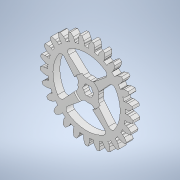
# Autodesk Inventor part: ｍ2歯数25ギア_6
Saved by Autodesk Inventor 2020.2 (Build 242310000, 310)
## iProperties
Created: 2020-03-11
Part Number: ｍ2歯数25ギア_6
Material: アルミニウム 2014-T4
Document SubType Name: Modeling
Designer: aoyam
Density: 2.8 g/cm^3
Appearance: サテン
Mass: 16.0283 g
Surface Area: 48.4557 cm^2
Volume: 5.70401 cm^3
Author: aoyam
Autodesk Inventor part; units mm, degrees
(part 1 of 2)
ref_plane "YZ Plane" through (0, 0, 0) normal (1, 0, 0) x (0, 1, 0)
ref_plane "XZ Plane" through (0, 0, 0) normal (0, 1, 0) x (-1, 0, 0)
ref_plane "XY Plane" through (0, 0, 0) normal (0, 0, 1) x (1, 0, 0)
sketch "スケッチ1" plane through (0, 0, 0) normal (0, 0, 1) x (1, 0, 0)
  arc A0 (2.4204, 26.4789) -> (2.3628, 26.1303) centre (4.6419, 25.9331) ccw
  arc A1 (2.7863, 27.5676) -> (2.4204, 26.4789) centre (8.5404, 25.0277) ccw
  arc A2 (3.906, 29.5327) -> (2.7863, 27.5676) centre (12.7407, 23.1969) ccw
  arc A3 (0.1118, 26.1303) -> (0.0542, 26.4789) centre (-2.1673, 25.9331) ccw
  arc A4 (0.0542, 26.4789) -> (-0.3117, 27.5676) centre (-6.0658, 25.0277) ccw
  arc A5 (-0.3117, 27.5676) -> (-1.4314, 29.5327) centre (-10.2661, 23.1969) ccw
  arc A6 (2.3153, 25.1391) -> (0.1593, 25.1391) centre (1.2373, 2.6649) ccw
  arc A7 (-1.4314, 29.5327) -> (-2.8596, 29.3523) centre (1.2373, 2.6649) ccw
  line L0 (2.3153, 25.1391) -> (2.3628, 26.1303)
  line L1 (0.1593, 25.1391) -> (0.1118, 26.1303)
  arc A8 (-3.5391, 26.0249) -> (-3.5082, 25.6729) centre (-1.2516, 26.0487) ccw
  line L2 (-3.3077, 24.7011) -> (-3.5082, 25.6729)
  arc A9 (-3.4554, 27.1705) -> (-3.5391, 26.0249) centre (2.7495, 26.1414) ccw
  arc A10 (-2.8596, 29.3523) -> (-3.4554, 27.1705) centre (7.2732, 25.4126) ccw
  arc A11 (-3.3077, 24.7011) -> (-5.3959, 24.1649) centre (1.2373, 2.6649) ccw
  line L3 (-5.3959, 24.1649) -> (-5.6884, 25.1131)
  arc A12 (-5.6884, 25.1131) -> (-5.8309, 25.4365) centre (-7.8469, 24.3554) ccw
  arc A13 (-6.4561, 26.4001) -> (-8.0293, 28.0249) centre (-15.0108, 19.691) ccw
  arc A14 (-8.0293, 28.0249) -> (-9.3677, 27.495) centre (1.2373, 2.6649) ccw
  arc A15 (-5.8309, 25.4365) -> (-6.4561, 26.4001) centre (-11.3978, 22.509) ccw
  arc A16 (-9.1985, 24.1032) -> (-9.0809, 23.77) centre (-6.9887, 24.6951) ccw
  line L4 (-8.6451, 22.8785) -> (-9.0809, 23.77)
  arc A17 (-9.4023, 25.2336) -> (-9.1985, 24.1032) centre (-3.1363, 25.7799) ccw
  arc A18 (-9.3677, 27.495) -> (-9.4023, 25.2336) centre (1.4265, 26.199) ccw
  arc A19 (-8.6451, 22.8785) -> (-10.5343, 21.8399) centre (1.2373, 2.6649) ccw
  line L5 (-10.5343, 21.8399) -> (-11.0535, 22.6855)
  arc A20 (-11.0535, 22.6855) -> (-11.2719, 22.9633) centre (-12.9557, 21.4148) ccw
  arc A21 (-12.1171, 23.7411) -> (-14.045, 24.9237) centre (-18.7346, 15.1154) ccw
  arc A22 (-14.045, 24.9237) -> (-15.2095, 24.0776) centre (1.2373, 2.6649) ccw
  arc A23 (-11.2719, 22.9633) -> (-12.1171, 23.7411) centre (-15.9358, 18.7433) ccw
  arc A24 (-14.2021, 20.8344) -> (-14.0054, 20.5409) centre (-12.209, 21.9573) ccw
  line L6 (-13.3615, 19.7858) -> (-14.0054, 20.5409)
  arc A25 (-14.6806, 21.8786) -> (-14.2021, 20.8344) centre (-8.7474, 23.966) ccw
  arc A26 (-15.2095, 24.0776) -> (-14.6806, 21.8786) centre (-4.4322, 25.5067) ccw
  arc A27 (-13.3615, 19.7858) -> (-14.9331, 18.31) centre (1.2373, 2.6649) ccw
  line L7 (-14.9331, 18.31) -> (-15.6463, 19)
  arc A28 (-15.6463, 19) -> (-15.9269, 19.2147) centre (-17.1727, 17.296) ccw
  arc A29 (-16.939, 19.7579) -> (-19.1004, 20.4238) centre (-21.2035, 9.7574) ccw
  arc A30 (-19.1004, 20.4238) -> (-20.0179, 19.3147) centre (1.2373, 2.6649) ccw
  arc A31 (-15.9269, 19.2147) -> (-16.939, 19.7579) centre (-19.3948, 13.9674) ccw
  arc A32 (-18.2356, 16.424) -> (-17.9721, 16.1886) centre (-16.5844, 18.0072) ccw
  line L8 (-17.1607, 15.6173) -> (-17.9721, 16.1886)
  arc A33 (-18.9588, 17.3163) -> (-18.2356, 16.424) centre (-13.7311, 20.8137) ccw
  arc A34 (-20.0179, 19.3147) -> (-18.9588, 17.3163) centre (-9.9346, 23.3792) ccw
  arc A35 (-17.1607, 15.6173) -> (-18.3159, 13.797) centre (1.2373, 2.6649) ccw
  line L9 (-18.3159, 13.797) -> (-19.1782, 14.288)
  arc A36 (-19.1782, 14.288) -> (-19.5034, 14.4262) centre (-20.2329, 12.258) ccw
  arc A37 (-20.6188, 14.7006) -> (-22.8779, 14.8081) centre (-22.2623, 3.9538) ccw
  arc A38 (-22.8779, 14.8081) -> (-23.4908, 13.5056) centre (1.2373, 2.6649) ccw
  arc A39 (-19.5034, 14.4262) -> (-20.6188, 14.7006) centre (-21.5575, 8.4813) ccw
  arc A40 (-21.0456, 11.149) -> (-20.7318, 10.9865) centre (-19.8399, 13.0932) ccw
  line L10 (-19.8038, 10.635) -> (-20.7318, 10.9865)
  arc A41 (-21.9679, 11.8335) -> (-21.0456, 11.149) centre (-17.7742, 16.5211) ccw
  arc A42 (-23.4908, 13.5056) -> (-21.9679, 11.8335) centre (-14.735, 19.9501) ccw
  arc A43 (-19.8038, 10.635) -> (-20.47, 8.5846) centre (1.2373, 2.6649) ccw
  line L11 (-20.47, 8.5846) -> (-21.4274, 8.8457)
  arc A44 (-21.4274, 8.8457) -> (-21.7767, 8.8987) centre (-21.9441, 6.6172) ccw
  arc A45 (-22.9253, 8.8871) -> (-25.1402, 8.4294) centre (-21.8445, -1.9308) ccw
  arc A46 (-25.1402, 8.4294) -> (-25.4099, 7.0154) centre (1.2373, 2.6649) ccw
  arc A47 (-21.7767, 8.8987) -> (-22.9253, 8.8871) centre (-22.2878, 2.6297) ccw
  arc A48 (-22.4554, 5.3409) -> (-22.1111, 5.2616) centre (-21.7712, 7.5238) ccw
  line L12 (-21.1248, 5.1519) -> (-22.1111, 5.2616)
  arc A49 (-23.519, 5.7745) -> (-22.4554, 5.3409) centre (-20.6228, 11.3578) ccw
  arc A50 (-25.4099, 7.0154) -> (-23.519, 5.7745) centre (-18.5318, 15.4349) ccw
  arc A51 (-21.1248, 5.1519) -> (-21.2602, 3.0002) centre (1.2373, 2.6649) ccw
  line L13 (-21.2602, 3.0002) -> (-22.2524, 3.015)
  arc A52 (-22.2524, 3.015) -> (-22.604, 2.9795) centre (-22.1987, 0.728) ccw
  arc A53 (-23.7136, 2.6826) -> (-25.745, 1.6885) centre (-19.9765, -7.5266) ccw
  arc A54 (-25.745, 1.6885) -> (-25.6547, 0.2519) centre (1.2373, 2.6649) ccw
  arc A55 (-22.604, 2.9795) -> (-23.7136, 2.6826) centre (-21.54, -3.2196) ccw
  arc A56 (-22.3766, -0.6353) -> (-22.0233, -0.6265) centre (-22.2567, 1.6492) ccw
  line L14 (-21.0408, -0.4875) -> (-22.0233, -0.6265)
  arc A57 (-23.5146, -0.4798) -> (-22.3766, -0.6353) centre (-22.0979, 5.6483) ccw
  arc A58 (-25.6547, 0.2519) -> (-23.5146, -0.4798) centre (-21.0865, 10.1173) ccw
  arc A59 (-21.0408, -0.4875) -> (-20.6368, -2.6052) centre (1.2373, 2.6649) ccw
  line L15 (-20.6368, -2.6052) -> (-21.6015, -2.8376)
  arc A60 (-21.6015, -2.8376) -> (-21.9332, -2.9595) centre (-20.9808, -5.0394) ccw
  arc A61 (-22.9341, -3.523) -> (-24.6545, -4.9911) centre (-16.7755, -12.4821) ccw
  arc A62 (-24.6545, -4.9911) -> (-24.2097, -6.3601) centre (1.2373, 2.6649) ccw
  arc A63 (-21.9332, -2.9595) -> (-22.9341, -3.523) centre (-19.361, -8.6992) ccw
  arc A64 (-20.814, -6.4041) -> (-20.474, -6.3078) centre (-21.266, -4.1616) ccw
  line L16 (-19.5569, -5.9288) -> (-20.474, -6.3078)
  arc A65 (-21.9549, -6.5366) -> (-20.814, -6.4041) centre (-22.1067, -0.2487) ccw
  arc A66 (-24.2097, -6.3601) -> (-21.9549, -6.5366) centre (-22.2385, 4.3315) ccw
  arc A67 (-19.5569, -5.9288) -> (-18.639, -7.8795) centre (1.2373, 2.6649) ccw
  line L17 (-18.639, -7.8795) -> (-19.5156, -8.3445)
  arc A68 (-19.5156, -8.3445) -> (-19.8065, -8.545) centre (-18.3667, -10.3228) ccw
  arc A69 (-20.6358, -9.3397) -> (-21.9371, -11.1896) centre (-12.4427, -16.4858) ccw
  arc A70 (-21.9371, -11.1896) -> (-21.1658, -12.405) centre (1.2373, 2.6649) ccw
  arc A71 (-19.8065, -8.545) -> (-20.6358, -9.3397) centre (-15.8877, -13.4648) ccw
  arc A72 (-17.8658, -11.6031) -> (-17.5605, -11.4252) centre (-18.8613, -9.5435) ccw
  line L18 (-16.7665, -10.8301) -> (-17.5605, -11.4252)
  arc A73 (-18.9379, -12.0152) -> (-17.8658, -11.6031) centre (-20.6487, -5.9626) ccw
  arc A74 (-21.1658, -12.405) -> (-18.9379, -12.0152) centre (-21.9154, -1.5591) ccw
  arc A75 (-16.7665, -10.8301) -> (-15.3922, -12.4912) centre (1.2373, 2.6649) ccw
  line L19 (-15.3922, -12.4912) -> (-16.1256, -13.1597)
  arc A76 (-16.1256, -13.1597) -> (-16.3576, -13.4262) centre (-14.5209, -14.7901) ccw
  arc A77 (-16.9632, -14.4022) -> (-17.7636, -16.5176) centre (-7.2503, -19.2862) ccw
  arc A78 (-17.7636, -16.5176) -> (-16.7142, -17.5029) centre (1.2373, 2.6649) ccw
  arc A79 (-16.3576, -13.4262) -> (-16.9632, -14.4022) centre (-11.3384, -17.2168) ccw
  arc A80 (-13.7173, -15.9056) -> (-13.4658, -15.6574) centre (-15.1938, -14.1582) ccw
  line L20 (-12.8448, -14.8835) -> (-13.4658, -15.6574)
  arc A81 (-14.6533, -16.5713) -> (-13.7173, -15.9056) centre (-17.8156, -11.1343) ccw
  arc A82 (-16.7142, -17.5029) -> (-14.6533, -16.5713) centre (-20.1376, -7.1842) ccw
  arc A83 (-12.8448, -14.8835) -> (-11.1006, -16.1507) centre (1.2373, 2.6649) ccw
  line L21 (-11.1006, -16.1507) -> (-11.6447, -16.9805)
  arc A84 (-11.6447, -16.9805) -> (-11.8031, -17.2964) centre (-9.685, -18.1606) ccw
  arc A85 (-12.147, -18.3923) -> (-12.3961, -20.6402) centre (-1.5246, -20.7074) ccw
  arc A86 (-12.3961, -20.6402) -> (-11.1347, -21.3337) centre (1.2373, 2.6649) ccw
  arc A87 (-11.8031, -17.2964) -> (-12.147, -18.3923) centre (-5.9989, -19.7197) ccw
  arc A88 (-8.6292, -19.0413) -> (-8.4473, -18.7383) centre (-10.4938, -17.7159) ccw
  line L22 (-8.0383, -17.8342) -> (-8.4473, -18.7383)
  arc A89 (-9.3702, -19.9188) -> (-8.6292, -19.0413) centre (-13.7853, -15.4391) ccw
  arc A90 (-11.1347, -21.3337) -> (-9.3702, -19.9188) centre (-17.0167, -12.1905) ccw
  arc A91 (-8.0383, -17.8342) -> (-6.0337, -18.6279) centre (1.2373, 2.6649) ccw
  line L23 (-6.0337, -18.6279) -> (-6.3544, -19.5669)
  arc A92 (-6.3544, -19.5669) -> (-6.4292, -19.9123) centre (-4.1627, -20.2226) ccw
  arc A93 (-6.4898, -21.0593) -> (-6.1721, -23.2986) centre (4.3746, -20.6599) ccw
  arc A94 (-6.1721, -23.2986) -> (-4.7778, -23.6565) centre (1.2373, 2.6649) ccw
  arc A95 (-6.4292, -19.9123) -> (-6.4898, -21.0593) centre (-0.2048, -20.816) ccw
  arc A96 (-2.9211, -20.813) -> (-2.8203, -20.4743) centre (-5.0567, -19.9931) ccw
  line L24 (-2.6489, -19.4969) -> (-2.8203, -20.4743)
  arc A97 (-3.4206, -21.8473) -> (-2.9211, -20.813) centre (-8.811, -18.6063) ccw
  arc A98 (-4.7778, -23.6565) -> (-3.4206, -21.8473) centre (-12.7488, -16.2634) ccw
  arc A99 (-2.6489, -19.4969) -> (-0.51, -19.7671) centre (1.2373, 2.6649) ccw
  line L25 (-0.51, -19.7671) -> (-0.5871, -20.7565)
  arc A100 (-0.5871, -20.7565) -> (-0.5737, -21.1096) centre (1.6988, -20.8465) ccw
  arc A101 (-0.3471, -22.2356) -> (0.5176, -24.3255) centre (10.0767, -19.1469) ccw
  arc A102 (0.5176, -24.3255) -> (1.957, -24.3255) centre (1.2373, 2.6649) ccw
  arc A103 (-0.5737, -21.1096) -> (-0.3471, -22.2356) centre (5.68, -20.4369) ccw
  arc A104 (3.0483, -21.1096) -> (3.0617, -20.7565) centre (0.7758, -20.8465) ccw
  line L26 (2.9846, -19.7671) -> (3.0617, -20.7565)
  arc A105 (2.8217, -22.2356) -> (3.0483, -21.1096) centre (-3.2054, -20.4369) ccw
  arc A106 (1.957, -24.3255) -> (2.8217, -22.2356) centre (-7.6021, -19.1469) ccw
  arc A107 (2.9846, -19.7671) -> (5.1235, -19.4969) centre (1.2373, 2.6649) ccw
  line L27 (5.1235, -19.4969) -> (5.2949, -20.4743)
  arc A108 (5.2949, -20.4743) -> (5.3957, -20.813) centre (7.5313, -19.9931) ccw
  arc A109 (5.8952, -21.8473) -> (7.2524, -23.6565) centre (15.2234, -16.2634) ccw
  arc A110 (7.2524, -23.6565) -> (8.6467, -23.2986) centre (1.2373, 2.6649) ccw
  arc A111 (5.3957, -20.813) -> (5.8952, -21.8473) centre (11.2856, -18.6063) ccw
  arc A112 (8.9038, -19.9123) -> (8.829, -19.5669) centre (6.6373, -20.2226) ccw
  line L28 (8.5083, -18.6279) -> (8.829, -19.5669)
  arc A113 (8.9644, -21.0593) -> (8.9038, -19.9123) centre (2.6794, -20.816) ccw
  arc A114 (8.6467, -23.2986) -> (8.9644, -21.0593) centre (-1.9, -20.6599) ccw
  arc A115 (8.5083, -18.6279) -> (10.5128, -17.8342) centre (1.2373, 2.6649) ccw
  line L29 (10.5128, -17.8342) -> (10.9219, -18.7383)
  arc A116 (10.9219, -18.7383) -> (11.1038, -19.0413) centre (12.9684, -17.7159) ccw
  arc A117 (11.8448, -19.9188) -> (13.6093, -21.3337) centre (19.4913, -12.1905) ccw
  arc A118 (13.6093, -21.3337) -> (14.8707, -20.6402) centre (1.2373, 2.6649) ccw
  arc A119 (11.1038, -19.0413) -> (11.8448, -19.9188) centre (16.2599, -15.4391) ccw
  arc A120 (14.2777, -17.2964) -> (14.1193, -16.9805) centre (12.1596, -18.1606) ccw
  line L30 (13.5752, -16.1507) -> (14.1193, -16.9805)
  arc A121 (14.6216, -18.3923) -> (14.2777, -17.2964) centre (8.4735, -19.7197) ccw
  arc A122 (14.8707, -20.6402) -> (14.6216, -18.3923) centre (3.9992, -20.7074) ccw
  arc A123 (13.5752, -16.1507) -> (15.3194, -14.8835) centre (1.2373, 2.6649) ccw
  line L31 (15.3194, -14.8835) -> (15.9404, -15.6574)
  arc A124 (15.9404, -15.6574) -> (16.1919, -15.9056) centre (17.6684, -14.1582) ccw
  arc A125 (17.1279, -16.5713) -> (19.1888, -17.5029) centre (22.6122, -7.1842) ccw
  arc A126 (19.1888, -17.5029) -> (20.2382, -16.5176) centre (1.2373, 2.6649) ccw
  arc A127 (16.1919, -15.9056) -> (17.1279, -16.5713) centre (20.2902, -11.1343) ccw
  arc A128 (18.8322, -13.4262) -> (18.6002, -13.1597) centre (16.9955, -14.7901) ccw
  line L32 (17.8668, -12.4912) -> (18.6002, -13.1597)
  arc A129 (19.4378, -14.4022) -> (18.8322, -13.4262) centre (13.813, -17.2168) ccw
  arc A130 (20.2382, -16.5176) -> (19.4378, -14.4022) centre (9.7249, -19.2862) ccw
  arc A131 (17.8668, -12.4912) -> (19.2411, -10.8301) centre (1.2373, 2.6649) ccw
  line L33 (19.2411, -10.8301) -> (20.0351, -11.4252)
  arc A132 (20.0351, -11.4252) -> (20.3404, -11.6031) centre (21.3359, -9.5435) ccw
  arc A133 (21.4125, -12.0152) -> (23.6404, -12.405) centre (24.39, -1.5591) ccw
  arc A134 (23.6404, -12.405) -> (24.4117, -11.1896) centre (1.2373, 2.6649) ccw
  arc A135 (20.3404, -11.6031) -> (21.4125, -12.0152) centre (23.1233, -5.9626) ccw
  arc A136 (22.2811, -8.545) -> (21.9902, -8.3445) centre (20.8413, -10.3228) ccw
  line L34 (21.1136, -7.8795) -> (21.9902, -8.3445)
  arc A137 (23.1104, -9.3397) -> (22.2811, -8.545) centre (18.3623, -13.4648) ccw
  arc A138 (24.4117, -11.1896) -> (23.1104, -9.3397) centre (14.9172, -16.4858) ccw
  arc A139 (21.1136, -7.8795) -> (22.0315, -5.9288) centre (1.2373, 2.6649) ccw
  line L35 (22.0315, -5.9288) -> (22.9486, -6.3078)
  arc A140 (22.9486, -6.3078) -> (23.2886, -6.4041) centre (23.7406, -4.1616) ccw
  arc A141 (24.4295, -6.5366) -> (26.6843, -6.3601) centre (24.7131, 4.3315) ccw
  arc A142 (26.6843, -6.3601) -> (27.1291, -4.9911) centre (1.2373, 2.6649) ccw
  arc A143 (23.2886, -6.4041) -> (24.4295, -6.5366) centre (24.5813, -0.2487) ccw
  arc A144 (24.4078, -2.9595) -> (24.0761, -2.8376) centre (23.4553, -5.0394) ccw
  line L36 (23.1114, -2.6052) -> (24.0761, -2.8376)
  arc A145 (25.4087, -3.523) -> (24.4078, -2.9595) centre (21.8356, -8.6992) ccw
  arc A146 (27.1291, -4.9911) -> (25.4087, -3.523) centre (19.2501, -12.4821) ccw
  arc A147 (23.1114, -2.6052) -> (23.5154, -0.4875) centre (1.2373, 2.6649) ccw
  line L37 (23.5154, -0.4875) -> (24.4979, -0.6265)
  arc A148 (24.4979, -0.6265) -> (24.8511, -0.6353) centre (24.7313, 1.6492) ccw
  arc A149 (25.9892, -0.4798) -> (28.1293, 0.2519) centre (23.5611, 10.1173) ccw
  arc A150 (28.1293, 0.2519) -> (28.2196, 1.6885) centre (1.2373, 2.6649) ccw
  arc A151 (24.8511, -0.6353) -> (25.9892, -0.4798) centre (24.5725, 5.6483) ccw
  arc A152 (25.0786, 2.9795) -> (24.727, 3.015) centre (24.6733, 0.728) ccw
  line L38 (23.7348, 3.0002) -> (24.727, 3.015)
  arc A153 (26.1881, 2.6826) -> (25.0786, 2.9795) centre (24.0146, -3.2196) ccw
  arc A154 (28.2196, 1.6885) -> (26.1881, 2.6826) centre (22.4511, -7.5266) ccw
  arc A155 (23.7348, 3.0002) -> (23.5994, 5.1519) centre (1.2373, 2.6649) ccw
  line L39 (23.5994, 5.1519) -> (24.5857, 5.2616)
  arc A156 (24.5857, 5.2616) -> (24.93, 5.3409) centre (24.2458, 7.5238) ccw
  arc A157 (25.9936, 5.7745) -> (27.8845, 7.0154) centre (21.0064, 15.4349) ccw
  arc A158 (27.8845, 7.0154) -> (27.6148, 8.4294) centre (1.2373, 2.6649) ccw
  arc A159 (24.93, 5.3409) -> (25.9936, 5.7745) centre (23.0974, 11.3578) ccw
  arc A160 (24.2513, 8.8987) -> (23.902, 8.8457) centre (24.4187, 6.6172) ccw
  line L40 (22.9446, 8.5846) -> (23.902, 8.8457)
  arc A161 (25.3999, 8.8871) -> (24.2513, 8.8987) centre (24.7624, 2.6297) ccw
  arc A162 (27.6148, 8.4294) -> (25.3999, 8.8871) centre (24.3191, -1.9308) ccw
  arc A163 (22.9446, 8.5846) -> (22.2784, 10.635) centre (1.2373, 2.6649) ccw
  line L41 (22.2784, 10.635) -> (23.2064, 10.9865)
  arc A164 (23.2064, 10.9865) -> (23.5202, 11.149) centre (22.3145, 13.0932) ccw
  arc A165 (24.4425, 11.8335) -> (25.9654, 13.5056) centre (17.2096, 19.9501) ccw
  arc A166 (25.9654, 13.5056) -> (25.3525, 14.8081) centre (1.2373, 2.6649) ccw
  arc A167 (23.5202, 11.149) -> (24.4425, 11.8335) centre (20.2488, 16.5211) ccw
  arc A168 (21.978, 14.4262) -> (21.6528, 14.288) centre (22.7075, 12.258) ccw
  line L42 (20.7905, 13.797) -> (21.6528, 14.288)
  arc A169 (23.0934, 14.7006) -> (21.978, 14.4262) centre (24.0321, 8.4813) ccw
  arc A170 (25.3525, 14.8081) -> (23.0934, 14.7006) centre (24.7369, 3.9538) ccw
  arc A171 (20.7905, 13.797) -> (19.6353, 15.6173) centre (1.2373, 2.6649) ccw
  line L43 (19.6353, 15.6173) -> (20.4467, 16.1886)
  arc A172 (20.4467, 16.1886) -> (20.7102, 16.424) centre (19.059, 18.0072) ccw
  arc A173 (21.4334, 17.3163) -> (22.4925, 19.3147) centre (12.4092, 23.3792) ccw
  arc A174 (22.4925, 19.3147) -> (21.575, 20.4238) centre (1.2373, 2.6649) ccw
  arc A175 (20.7102, 16.424) -> (21.4334, 17.3163) centre (16.2057, 20.8137) ccw
  arc A176 (18.4015, 19.2147) -> (18.1209, 19) centre (19.6473, 17.296) ccw
  line L44 (17.4077, 18.31) -> (18.1209, 19)
  arc A177 (19.4136, 19.7579) -> (18.4015, 19.2147) centre (21.8694, 13.9674) ccw
  arc A178 (21.575, 20.4238) -> (19.4136, 19.7579) centre (23.678, 9.7574) ccw
  arc A179 (17.4077, 18.31) -> (15.8361, 19.7858) centre (1.2373, 2.6649) ccw
  line L45 (15.8361, 19.7858) -> (16.48, 20.5409)
  arc A180 (16.48, 20.5409) -> (16.6767, 20.8344) centre (14.6836, 21.9573) ccw
  arc A181 (17.1552, 21.8786) -> (17.6841, 24.0776) centre (6.9067, 25.5067) ccw
  arc A182 (17.6841, 24.0776) -> (16.5196, 24.9237) centre (1.2373, 2.6649) ccw
  arc A183 (16.6767, 20.8344) -> (17.1552, 21.8786) centre (11.222, 23.966) ccw
  arc A184 (13.7465, 22.9633) -> (13.5281, 22.6855) centre (15.4303, 21.4148) ccw
  line L46 (13.0089, 21.8399) -> (13.5281, 22.6855)
  arc A185 (14.5917, 23.7411) -> (13.7465, 22.9633) centre (18.4104, 18.7433) ccw
  arc A186 (16.5196, 24.9237) -> (14.5917, 23.7411) centre (21.2092, 15.1154) ccw
  arc A187 (13.0089, 21.8399) -> (11.1197, 22.8785) centre (1.2373, 2.6649) ccw
  line L47 (11.1197, 22.8785) -> (11.5555, 23.77)
  arc A188 (11.5555, 23.77) -> (11.6731, 24.1032) centre (9.4633, 24.6951) ccw
  arc A189 (11.8769, 25.2336) -> (11.8423, 27.495) centre (1.0481, 26.199) ccw
  arc A190 (11.8423, 27.495) -> (10.5039, 28.0249) centre (1.2373, 2.6649) ccw
  arc A191 (11.6731, 24.1032) -> (11.8769, 25.2336) centre (5.6109, 25.7799) ccw
  arc A192 (8.3055, 25.4365) -> (8.163, 25.1131) centre (10.3215, 24.3554) ccw
  line L48 (7.8705, 24.1649) -> (8.163, 25.1131)
  arc A193 (8.9307, 26.4001) -> (8.3055, 25.4365) centre (13.8724, 22.509) ccw
  arc A194 (10.5039, 28.0249) -> (8.9307, 26.4001) centre (17.4854, 19.691) ccw
  arc A195 (7.8705, 24.1649) -> (5.7823, 24.7011) centre (1.2373, 2.6649) ccw
  line L49 (5.7823, 24.7011) -> (5.9828, 25.6729)
  arc A196 (5.9828, 25.6729) -> (6.0137, 26.0249) centre (3.7262, 26.0487) ccw
  arc A197 (5.93, 27.1705) -> (5.3342, 29.3523) centre (-4.7987, 25.4126) ccw
  arc A198 (5.3342, 29.3523) -> (3.906, 29.5327) centre (1.2373, 2.6649) ccw
  arc A199 (6.0137, 26.0249) -> (5.93, 27.1705) centre (-0.275, 26.1414) ccw
  line L50 (3.9047, 1.785) -> (3.322, 0.7756)
  line L51 (1.8089, -0.0851) -> (0.6435, -0.0851)
  line L52 (-0.8585, 0.7949) -> (-1.4412, 1.8042)
  line L53 (-1.4301, 3.5449) -> (-0.8474, 4.5542)
  line L54 (3.333, 4.535) -> (3.9158, 3.5256)
  line L55 (1.2373, 2.6649) -> (-0.3396, 5.4149) construction
  arc A200 (0.6657, 5.4149) -> (-0.8474, 4.5542) centre (0.1576, 4.5478) ccw
  arc A201 (-1.4301, 3.5449) -> (-1.4412, 1.8042) centre (-0.9331, 2.6713) ccw
  arc A202 (-0.8585, 0.7949) -> (0.6435, -0.0851) centre (0.1465, 0.7885) ccw
  arc A203 (1.8089, -0.0851) -> (3.322, 0.7756) centre (2.317, 0.782) ccw
  arc A204 (3.9047, 1.785) -> (3.9158, 3.5256) centre (3.4077, 2.6585) ccw
  arc A205 (3.333, 4.535) -> (1.8311, 5.4149) centre (2.3281, 4.5414) ccw
  line L56 (-0.3504, 5.4149) -> (-0.3396, 5.4149)
  line L57 (0.6657, 5.4149) -> (1.8311, 5.4149)
  circle A206 centre (1.2373, 2.6649) radius 22.5
  circle A207 centre (1.2373, 2.6649) radius 6
  circle A208 centre (1.2373, 2.6649) radius 19.5
  line L58 (1.2373, 2.6649) -> (-12.1169, 16.8746)
  line L59 (-4.3198, 4.9275) -> (-13.1696, 15.8061)
  line L60 (-0.6762, 8.3516) -> (-10.9851, 17.8591)
  line L61 (-1.0252, -2.8921) -> (-11.9039, -11.742)
  line L62 (-4.4494, 0.7514) -> (-13.9569, -9.5575)
  line L63 (6.7944, 0.4024) -> (15.6442, -10.4763)
  line L64 (3.1508, -3.0218) -> (13.4597, -12.5293)
  line L65 (3.4998, 8.222) -> (14.3785, 17.0718)
  line L66 (6.924, 4.5784) -> (16.4315, 14.8873)
  point P0 (0, 0)
  point P1 (-1.9381, 2.6649)
  point P2 (-0.3504, -0.0851)
  point P3 (2.825, -0.0851)
  point P4 (4.4127, 2.6649)
  point P5 (2.825, 5.4149)
  point P6 (6.0137, 26.0249)
  point P7 (5.93, 27.1705)
  point P8 (5.3342, 29.3523)
  point P9 (3.906, 29.5327)
  point P10 (2.7863, 27.5676)
  point P11 (2.4204, 26.4789)
  point P12 (2.3153, 25.1391)
  point P13 (0.0542, 26.4789)
  point P14 (-0.3117, 27.5676)
  point P15 (-2.8596, 29.3523)
  point P16 (-3.4554, 27.1705)
  point P17 (-3.5391, 26.0249)
  point P18 (-3.3077, 24.7011)
  point P19 (-5.3959, 24.1649)
  point P20 (-5.8309, 25.4365)
  point P21 (-6.4561, 26.4001)
  point P22 (-9.3677, 27.495)
  point P23 (-9.0809, 23.77)
  point P24 (-8.6451, 22.8785)
  point P25 (-10.5343, 21.8399)
  point P26 (-11.2719, 22.9633)
  point P27 (-12.1171, 23.7411)
  point P28 (-15.2095, 24.0776)
  point P29 (-14.2021, 20.8344)
  point P30 (-14.0054, 20.5409)
  point P31 (-13.3615, 19.7858)
  point P32 (-14.9331, 18.31)
  point P33 (-15.6463, 19)
  point P34 (-15.9269, 19.2147)
  point P35 (-16.939, 19.7579)
  point P36 (-19.1004, 20.4238)
  point P37 (-20.0179, 19.3147)
  point P38 (-18.9588, 17.3163)
  point P39 (-18.2356, 16.424)
  point P40 (-17.9721, 16.1886)
  point P41 (-19.5034, 14.4262)
  point P42 (-20.6188, 14.7006)
  point P43 (-22.8779, 14.8081)
  point P44 (-23.4908, 13.5056)
  point P45 (-21.9679, 11.8335)
  point P46 (-21.0456, 11.149)
  point P47 (-20.7318, 10.9865)
  point P48 (-19.8038, 10.635)
  point P49 (-21.4274, 8.8457)
  point P50 (-21.7767, 8.8987)
  point P51 (-22.9253, 8.8871)
  point P52 (-25.1402, 8.4294)
  point P53 (-25.4099, 7.0154)
  point P54 (-23.519, 5.7745)
  point P55 (-22.4554, 5.3409)
  point P56 (-22.604, 2.9795)
  point P57 (-23.7136, 2.6826)
  point P58 (-25.6547, 0.2519)
  point P59 (-23.5146, -0.4798)
  point P60 (-22.3766, -0.6353)
  point P61 (-21.9332, -2.9595)
  point P62 (-22.9341, -3.523)
  point P63 (-24.6545, -4.9911)
  point P64 (-24.2097, -6.3601)
  point P65 (-21.9549, -6.5366)
  point P66 (-20.814, -6.4041)
  point P67 (-19.5569, -5.9288)
  point P68 (-18.639, -7.8795)
  point P69 (-19.8065, -8.545)
  point P70 (-20.6358, -9.3397)
  point P71 (-21.9371, -11.1896)
  point P72 (-21.1658, -12.405)
  point P73 (-17.8658, -11.6031)
  point P74 (-17.5605, -11.4252)
  point P75 (-16.7665, -10.8301)
  point P76 (-16.3576, -13.4262)
  point P77 (-17.7636, -16.5176)
  point P78 (-16.7142, -17.5029)
  point P79 (-13.7173, -15.9056)
  point P80 (-11.6447, -16.9805)
  point P81 (-11.8031, -17.2964)
  point P82 (-12.147, -18.3923)
  point P83 (-11.1347, -21.3337)
  point P84 (-9.3702, -19.9188)
  point P85 (-8.6292, -19.0413)
  point P86 (-8.4473, -18.7383)
  point P87 (-6.3544, -19.5669)
  point P88 (-6.4292, -19.9123)
  point P89 (-6.4898, -21.0593)
  point P90 (-4.7778, -23.6565)
  point P91 (-3.4206, -21.8473)
  point P92 (-2.9211, -20.813)
  point P93 (-2.6489, -19.4969)
  point P94 (-0.51, -19.7671)
  point P95 (-0.5737, -21.1096)
  point P96 (-0.3471, -22.2356)
  point P97 (0.5176, -24.3255)
  point P98 (1.957, -24.3255)
  point P99 (2.8217, -22.2356)
  point P100 (3.0483, -21.1096)
  point P101 (5.1235, -19.4969)
  point P102 (5.2949, -20.4743)
  point P103 (5.3957, -20.813)
  point P104 (5.8952, -21.8473)
  point P105 (7.2524, -23.6565)
  point P106 (8.6467, -23.2986)
  point P107 (8.9644, -21.0593)
  point P108 (8.9038, -19.9123)
  point P109 (8.829, -19.5669)
  point P110 (8.5083, -18.6279)
  point P111 (11.1038, -19.0413)
  point P112 (11.8448, -19.9188)
  point P113 (13.6093, -21.3337)
  point P114 (14.8707, -20.6402)
  point P115 (14.6216, -18.3923)
  point P116 (14.2777, -17.2964)
  point P117 (13.5752, -16.1507)
  point P118 (15.3194, -14.8835)
  point P119 (16.1919, -15.9056)
  point P120 (17.1279, -16.5713)
  point P121 (19.1888, -17.5029)
  point P122 (20.2382, -16.5176)
  point P123 (19.4378, -14.4022)
  point P124 (18.8322, -13.4262)
  point P125 (19.2411, -10.8301)
  point P126 (20.0351, -11.4252)
  point P127 (20.3404, -11.6031)
  point P128 (21.4125, -12.0152)
  point P129 (24.4117, -11.1896)
  point P130 (23.1104, -9.3397)
  point P131 (22.2811, -8.545)
  point P132 (21.1136, -7.8795)
  point P133 (22.0315, -5.9288)
  point P134 (23.2886, -6.4041)
  point P135 (24.4295, -6.5366)
  point P136 (26.6843, -6.3601)
  point P137 (27.1291, -4.9911)
  point P138 (24.4078, -2.9595)
  point P139 (24.0761, -2.8376)
  point P140 (23.1114, -2.6052)
  point P141 (24.8511, -0.6353)
  point P142 (25.9892, -0.4798)
  point P143 (28.1293, 0.2519)
  point P144 (28.2196, 1.6885)
  point P145 (26.1881, 2.6826)
  point P146 (25.0786, 2.9795)
  point P147 (24.727, 3.015)
  point P148 (23.7348, 3.0002)
  point P149 (24.93, 5.3409)
  point P150 (25.9936, 5.7745)
  point P151 (27.6148, 8.4294)
  point P152 (25.3999, 8.8871)
  point P153 (24.2513, 8.8987)
  point P154 (23.902, 8.8457)
  point P155 (22.9446, 8.5846)
  point P156 (23.2064, 10.9865)
  point P157 (23.5202, 11.149)
  point P158 (24.4425, 11.8335)
  point P159 (25.9654, 13.5056)
  point P160 (25.3525, 14.8081)
  point P161 (23.0934, 14.7006)
  point P162 (21.978, 14.4262)
  point P163 (19.6353, 15.6173)
  point P164 (20.4467, 16.1886)
  point P165 (20.7102, 16.424)
  point P166 (21.4334, 17.3163)
  point P167 (22.4925, 19.3147)
  point P168 (21.575, 20.4238)
  point P169 (19.4136, 19.7579)
  point P170 (18.4015, 19.2147)
  point P171 (18.1209, 19)
  point P172 (16.48, 20.5409)
  point P173 (16.6767, 20.8344)
  point P174 (17.1552, 21.8786)
  point P175 (17.6841, 24.0776)
  point P176 (16.5196, 24.9237)
  point P177 (14.5917, 23.7411)
  point P178 (13.7465, 22.9633)
  point P179 (13.0089, 21.8399)
  point P180 (11.1197, 22.8785)
  point P181 (11.5555, 23.77)
  point P182 (11.6731, 24.1032)
  point P183 (11.8769, 25.2336)
  point P184 (11.8423, 27.495)
  point P185 (10.5039, 28.0249)
  point P186 (8.3055, 25.4365)
  point P187 (8.163, 25.1131)
  point P188 (-0.6762, 8.3516)
  point P189 (3.4998, 8.222)
  point P190 (6.7944, 0.4024)
  point P191 (6.924, 4.5784)
  point P192 (-1.0252, -2.8921)
  point P193 (3.1508, -3.0218)
  point P194 (13.4597, -12.5293)
  point P195 (-11.9039, -11.742)
  point P196 (-4.4494, 0.7514)
  point P197 (-13.9569, -9.5575)
  dimension "d2" = 360
  dimension "d5" = 2.01
  dimension "d8" = 360
  dimension "d13" = 3
  dimension "d14" = 1.5
  dimension "d17" = 360
  dimension "d23" = 2.5
  constraints: 420 point on circle, 207 centre point, 134 end point, 5 coincident, 2 horizontal, 2 symmetric about line, 1 point on line, 1017 other
  measures "d5" diameter of A200
  measures "d14" distance of L58.end L59.end
  measures "d23" distance from line of L58 L59.start
extrude "押し出し1" add sketch "スケッチ1" along normal blind 4 contours A1 A2 A198 A197 A199 A196 L49 A206 L0 A0 | A206 A195 A187 A179 A171 A163 A155 A147 A139 A131 A123 A115 A107 A99 A91 A83 A75 A67 A59 A51 A43 A35 A27 A19 A11 A6 | A206 L2 A8 A9 A10 A7 A5 A4 A3 L1 | L48 A192 A193 A194 A190 A189 A191 A188 L47 A206 | A206 L4 A16 A17 A18 A14 A13 A15 A12 L3 | L46 A184 A185 A186 A182 A181 A183 A180 L45 A206 | A206 L6 A24 A25 A26 A22 A21 A23 A20 L5 | L44 A176 A177 A178 A174 A173 A175 A172 L43 A206 | A206 L8 A32 A33 A34 A30 A29 A31 A28 L7 | L42 A168 A169 A170 A166 A165 A167 A164 L41 A206 | A206 L10 A40 A41 A42 A38 A37 A39 A36 L9 | L40 A160 A161 A162 A158 A157 A159 A156 L39 A206 | A206 L12 A48 A49 A50 A46 A45 A47 A44 L11 | L38 A152 A153 A154 A150 A149 A151 A148 L37 A206 | A206 L14 A56 A57 A58 A54 A53 A55 A52 L13 | A206 L16 A64 A65 A66 A62 A61 A63 A60 L15 | L36 A144 A145 A146 A142 A141 A143 A140 L35 A206 | A206 L18 A72 A73 A74 A70 A69 A71 A68 L17 | L34 A136 A137 A138 A134 A133 A135 A132 L33 A206 | A206 L20 A80 A81 A82 A78 A77 A79 A76 L19 | L32 A128 A129 A130 A126 A125 A127 A124 L31 A206 | A206 L22 A88 A89 A90 A86 A85 A87 A84 L21 | L30 A120 A121 A122 A118 A117 A119 A116 L29 A206 | A206 L24 A96 A97 A98 A94 A93 A95 A92 L23 | L28 A112 A113 A114 A110 A109 A111 A108 L27 A206 | A206 L26 A104 A105 A106 A102 A101 A103 A100 L25 | A207 | A207 L65 A208 L66 | L63 A208 L64 A207 | A207 L58 A208 L60 | L61 A208 L62 A207 | A207 L59 A208 L58
fillet "フィレット1" radius 2.1 16 edges at (-10.9851, 17.8591, 2) (3.4998, 8.222, 2) (-0.6762, 8.3516, 2) (14.3785, 17.0718, 2) (6.924, 4.5784, 2) (6.7944, 0.4024, 2) (15.6442, -10.4763, 2) (16.4315, 14.8873, 2) (13.4597, -12.5293, 2) (3.1508, -3.0218, 2) (-1.0252, -2.8921, 2) (-11.9039, -11.742, 2) (-4.3198, 4.9275, 2) (-4.4494, 0.7514, 2) (-13.9569, -9.5575, 2) (-13.1696, 15.8061, 2)
sketch "スケッチ3" plane through (0, 0, 4) normal (0, 0, 1) x (1, 0, 0)
  arc A0 (20.4467, 16.1886) -> (20.7102, 16.424) centre (19.059, 18.0072) ccw projected
  arc A1 (20.7102, 16.424) -> (21.4334, 17.3163) centre (16.2057, 20.8137) ccw projected
  arc A2 (21.4334, 17.3163) -> (22.4925, 19.3147) centre (12.4092, 23.3792) ccw projected
  arc A3 (22.4925, 19.3147) -> (21.575, 20.4238) centre (1.2373, 2.6649) ccw projected
  arc A4 (21.575, 20.4238) -> (19.4136, 19.7579) centre (23.678, 9.7574) ccw projected
  arc A5 (19.4136, 19.7579) -> (18.4015, 19.2147) centre (21.8694, 13.9674) ccw projected
  arc A6 (18.4015, 19.2147) -> (18.1209, 19) centre (19.6473, 17.296) ccw projected
  line L0 (18.1209, 19) -> (17.4077, 18.31) projected
  arc A7 (17.4077, 18.31) -> (15.8361, 19.7858) centre (1.2373, 2.6649) ccw projected
  line L1 (15.8361, 19.7858) -> (16.48, 20.5409) projected
  arc A8 (16.48, 20.5409) -> (16.6767, 20.8344) centre (14.6836, 21.9573) ccw projected
  arc A9 (16.6767, 20.8344) -> (17.1552, 21.8786) centre (11.222, 23.966) ccw projected
  arc A10 (17.1552, 21.8786) -> (17.6841, 24.0776) centre (6.9067, 25.5067) ccw projected
  arc A11 (17.6841, 24.0776) -> (16.5196, 24.9237) centre (1.2373, 2.6649) ccw projected
  arc A12 (16.5196, 24.9237) -> (14.5917, 23.7411) centre (21.2092, 15.1154) ccw projected
  arc A13 (14.5917, 23.7411) -> (13.7465, 22.9633) centre (18.4104, 18.7433) ccw projected
  arc A14 (13.7465, 22.9633) -> (13.5281, 22.6855) centre (15.4303, 21.4148) ccw projected
  line L2 (13.5281, 22.6855) -> (13.0089, 21.8399) projected
  arc A15 (13.0089, 21.8399) -> (11.1197, 22.8785) centre (1.2373, 2.6649) ccw projected
  line L3 (11.1197, 22.8785) -> (11.5555, 23.77) projected
  arc A16 (11.5555, 23.77) -> (11.6731, 24.1032) centre (9.4633, 24.6951) ccw projected
  arc A17 (11.6731, 24.1032) -> (11.8769, 25.2336) centre (5.6109, 25.7799) ccw projected
  arc A18 (11.8769, 25.2336) -> (11.8423, 27.495) centre (1.0481, 26.199) ccw projected
  arc A19 (11.8423, 27.495) -> (10.5039, 28.0249) centre (1.2373, 2.6649) ccw projected
  arc A20 (10.5039, 28.0249) -> (8.9307, 26.4001) centre (17.4854, 19.691) ccw projected
  arc A21 (8.9307, 26.4001) -> (8.3055, 25.4365) centre (13.8724, 22.509) ccw projected
  arc A22 (8.3055, 25.4365) -> (8.163, 25.1131) centre (10.3215, 24.3554) ccw projected
  line L4 (8.163, 25.1131) -> (7.8705, 24.1649) projected
  arc A23 (7.8705, 24.1649) -> (5.7823, 24.7011) centre (1.2373, 2.6649) ccw projected
  line L5 (5.7823, 24.7011) -> (5.9828, 25.6729) projected
  arc A24 (5.9828, 25.6729) -> (6.0137, 26.0249) centre (3.7262, 26.0487) ccw projected
  arc A25 (6.0137, 26.0249) -> (5.93, 27.1705) centre (-0.275, 26.1414) ccw projected
  arc A26 (5.93, 27.1705) -> (5.3342, 29.3523) centre (-4.7987, 25.4126) ccw projected
  arc A27 (5.3342, 29.3523) -> (3.906, 29.5327) centre (1.2373, 2.6649) ccw projected
  arc A28 (3.906, 29.5327) -> (2.7863, 27.5676) centre (12.7407, 23.1969) ccw projected
  arc A29 (2.7863, 27.5676) -> (2.4204, 26.4789) centre (8.5404, 25.0277) ccw projected
  arc A30 (2.4204, 26.4789) -> (2.3628, 26.1303) centre (4.6419, 25.9331) ccw projected
  line L6 (2.3628, 26.1303) -> (2.3153, 25.1391) projected
  arc A31 (2.3153, 25.1391) -> (0.1593, 25.1391) centre (1.2373, 2.6649) ccw projected
  line L7 (0.1593, 25.1391) -> (0.1118, 26.1303) projected
  arc A32 (0.1118, 26.1303) -> (0.0542, 26.4789) centre (-2.1673, 25.9331) ccw projected
  arc A33 (0.0542, 26.4789) -> (-0.3117, 27.5676) centre (-6.0658, 25.0277) ccw projected
  arc A34 (-0.3117, 27.5676) -> (-1.4314, 29.5327) centre (-10.2661, 23.1969) ccw projected
  arc A35 (-1.4314, 29.5327) -> (-2.8596, 29.3523) centre (1.2373, 2.6649) ccw projected
  arc A36 (-2.8596, 29.3523) -> (-3.4554, 27.1705) centre (7.2732, 25.4126) ccw projected
  arc A37 (-3.4554, 27.1705) -> (-3.5391, 26.0249) centre (2.7495, 26.1414) ccw projected
  arc A38 (-3.5391, 26.0249) -> (-3.5082, 25.6729) centre (-1.2516, 26.0487) ccw projected
  line L8 (-3.5082, 25.6729) -> (-3.3077, 24.7011) projected
  arc A39 (-3.3077, 24.7011) -> (-5.3959, 24.1649) centre (1.2373, 2.6649) ccw projected
  line L9 (-5.3959, 24.1649) -> (-5.6884, 25.1131) projected
  arc A40 (-5.6884, 25.1131) -> (-5.8309, 25.4365) centre (-7.8469, 24.3554) ccw projected
  arc A41 (-5.8309, 25.4365) -> (-6.4561, 26.4001) centre (-11.3978, 22.509) ccw projected
  arc A42 (-6.4561, 26.4001) -> (-8.0293, 28.0249) centre (-15.0108, 19.691) ccw projected
  arc A43 (-8.0293, 28.0249) -> (-9.3677, 27.495) centre (1.2373, 2.6649) ccw projected
  arc A44 (-9.3677, 27.495) -> (-9.4023, 25.2336) centre (1.4265, 26.199) ccw projected
  arc A45 (-9.4023, 25.2336) -> (-9.1985, 24.1032) centre (-3.1363, 25.7799) ccw projected
  arc A46 (-9.1985, 24.1032) -> (-9.0809, 23.77) centre (-6.9887, 24.6951) ccw projected
  line L10 (-9.0809, 23.77) -> (-8.6451, 22.8785) projected
  arc A47 (-8.6451, 22.8785) -> (-10.5343, 21.8399) centre (1.2373, 2.6649) ccw projected
  line L11 (-10.5343, 21.8399) -> (-11.0535, 22.6855) projected
  arc A48 (-11.0535, 22.6855) -> (-11.2719, 22.9633) centre (-12.9557, 21.4148) ccw projected
  arc A49 (-11.2719, 22.9633) -> (-12.1171, 23.7411) centre (-15.9358, 18.7433) ccw projected
  arc A50 (-12.1171, 23.7411) -> (-14.045, 24.9237) centre (-18.7346, 15.1154) ccw projected
  arc A51 (-14.045, 24.9237) -> (-15.2095, 24.0776) centre (1.2373, 2.6649) ccw projected
  arc A52 (-15.2095, 24.0776) -> (-14.6806, 21.8786) centre (-4.4322, 25.5067) ccw projected
  arc A53 (-14.6806, 21.8786) -> (-14.2021, 20.8344) centre (-8.7474, 23.966) ccw projected
  arc A54 (-14.2021, 20.8344) -> (-14.0054, 20.5409) centre (-12.209, 21.9573) ccw projected
  line L12 (-14.0054, 20.5409) -> (-13.3615, 19.7858) projected
  arc A55 (-13.3615, 19.7858) -> (-14.9331, 18.31) centre (1.2373, 2.6649) ccw projected
  line L13 (-14.9331, 18.31) -> (-15.6463, 19) projected
  arc A56 (-15.6463, 19) -> (-15.9269, 19.2147) centre (-17.1727, 17.296) ccw projected
  arc A57 (-15.9269, 19.2147) -> (-16.939, 19.7579) centre (-19.3948, 13.9674) ccw projected
  arc A58 (-16.939, 19.7579) -> (-19.1004, 20.4238) centre (-21.2035, 9.7574) ccw projected
  arc A59 (-19.1004, 20.4238) -> (-20.0179, 19.3147) centre (1.2373, 2.6649) ccw projected
  arc A60 (-20.0179, 19.3147) -> (-18.9588, 17.3163) centre (-9.9346, 23.3792) ccw projected
  arc A61 (-18.9588, 17.3163) -> (-18.2356, 16.424) centre (-13.7311, 20.8137) ccw projected
  arc A62 (-18.2356, 16.424) -> (-17.9721, 16.1886) centre (-16.5844, 18.0072) ccw projected
  line L14 (-17.9721, 16.1886) -> (-17.1607, 15.6173) projected
  arc A63 (-17.1607, 15.6173) -> (-18.3159, 13.797) centre (1.2373, 2.6649) ccw projected
  line L15 (-18.3159, 13.797) -> (-19.1782, 14.288) projected
  arc A64 (-19.1782, 14.288) -> (-19.5034, 14.4262) centre (-20.2329, 12.258) ccw projected
  arc A65 (-19.5034, 14.4262) -> (-20.6188, 14.7006) centre (-21.5575, 8.4813) ccw projected
  arc A66 (-20.6188, 14.7006) -> (-22.8779, 14.8081) centre (-22.2623, 3.9538) ccw projected
  arc A67 (-22.8779, 14.8081) -> (-23.4908, 13.5056) centre (1.2373, 2.6649) ccw projected
  arc A68 (-23.4908, 13.5056) -> (-21.9679, 11.8335) centre (-14.735, 19.9501) ccw projected
  arc A69 (-21.9679, 11.8335) -> (-21.0456, 11.149) centre (-17.7742, 16.5211) ccw projected
  arc A70 (-21.0456, 11.149) -> (-20.7318, 10.9865) centre (-19.8399, 13.0932) ccw projected
  line L16 (-20.7318, 10.9865) -> (-19.8038, 10.635) projected
  arc A71 (-19.8038, 10.635) -> (-20.47, 8.5846) centre (1.2373, 2.6649) ccw projected
  line L17 (-20.47, 8.5846) -> (-21.4274, 8.8457) projected
  arc A72 (-21.4274, 8.8457) -> (-21.7767, 8.8987) centre (-21.9441, 6.6172) ccw projected
  arc A73 (-21.7767, 8.8987) -> (-22.9253, 8.8871) centre (-22.2878, 2.6297) ccw projected
  arc A74 (-22.9253, 8.8871) -> (-25.1402, 8.4294) centre (-21.8445, -1.9308) ccw projected
  arc A75 (-25.1402, 8.4294) -> (-25.4099, 7.0154) centre (1.2373, 2.6649) ccw projected
  arc A76 (-25.4099, 7.0154) -> (-23.519, 5.7745) centre (-18.5318, 15.4349) ccw projected
  arc A77 (-23.519, 5.7745) -> (-22.4554, 5.3409) centre (-20.6228, 11.3578) ccw projected
  arc A78 (-22.4554, 5.3409) -> (-22.1111, 5.2616) centre (-21.7712, 7.5238) ccw projected
  line L18 (-22.1111, 5.2616) -> (-21.1248, 5.1519) projected
  arc A79 (-21.1248, 5.1519) -> (-21.2602, 3.0002) centre (1.2373, 2.6649) ccw projected
  line L19 (-21.2602, 3.0002) -> (-22.2524, 3.015) projected
  arc A80 (-22.2524, 3.015) -> (-22.604, 2.9795) centre (-22.1987, 0.728) ccw projected
  arc A81 (-22.604, 2.9795) -> (-23.7136, 2.6826) centre (-21.54, -3.2196) ccw projected
  arc A82 (-23.7136, 2.6826) -> (-25.745, 1.6885) centre (-19.9765, -7.5266) ccw projected
  arc A83 (-25.745, 1.6885) -> (-25.6547, 0.2519) centre (1.2373, 2.6649) ccw projected
  arc A84 (-25.6547, 0.2519) -> (-23.5146, -0.4798) centre (-21.0865, 10.1173) ccw projected
  arc A85 (-23.5146, -0.4798) -> (-22.3766, -0.6353) centre (-22.0979, 5.6483) ccw projected
  arc A86 (-22.3766, -0.6353) -> (-22.0233, -0.6265) centre (-22.2567, 1.6492) ccw projected
  line L20 (-22.0233, -0.6265) -> (-21.0408, -0.4875) projected
  arc A87 (-21.0408, -0.4875) -> (-20.6368, -2.6052) centre (1.2373, 2.6649) ccw projected
  line L21 (-20.6368, -2.6052) -> (-21.6015, -2.8376) projected
  arc A88 (-21.6015, -2.8376) -> (-21.9332, -2.9595) centre (-20.9808, -5.0394) ccw projected
  arc A89 (-21.9332, -2.9595) -> (-22.9341, -3.523) centre (-19.361, -8.6992) ccw projected
  arc A90 (-22.9341, -3.523) -> (-24.6545, -4.9911) centre (-16.7755, -12.4821) ccw projected
  arc A91 (-24.6545, -4.9911) -> (-24.2097, -6.3601) centre (1.2373, 2.6649) ccw projected
  arc A92 (-24.2097, -6.3601) -> (-21.9549, -6.5366) centre (-22.2385, 4.3315) ccw projected
  arc A93 (-21.9549, -6.5366) -> (-20.814, -6.4041) centre (-22.1067, -0.2487) ccw projected
  arc A94 (-20.814, -6.4041) -> (-20.474, -6.3078) centre (-21.266, -4.1616) ccw projected
  line L22 (-20.474, -6.3078) -> (-19.5569, -5.9288) projected
  arc A95 (-19.5569, -5.9288) -> (-18.639, -7.8795) centre (1.2373, 2.6649) ccw projected
  line L23 (-18.639, -7.8795) -> (-19.5156, -8.3445) projected
  arc A96 (-19.5156, -8.3445) -> (-19.8065, -8.545) centre (-18.3667, -10.3228) ccw projected
  arc A97 (-19.8065, -8.545) -> (-20.6358, -9.3397) centre (-15.8877, -13.4648) ccw projected
  arc A98 (-20.6358, -9.3397) -> (-21.9371, -11.1896) centre (-12.4427, -16.4858) ccw projected
  arc A99 (-21.9371, -11.1896) -> (-21.1658, -12.405) centre (1.2373, 2.6649) ccw projected
  arc A100 (-21.1658, -12.405) -> (-18.9379, -12.0152) centre (-21.9154, -1.5591) ccw projected
  arc A101 (-18.9379, -12.0152) -> (-17.8658, -11.6031) centre (-20.6487, -5.9626) ccw projected
  arc A102 (-17.8658, -11.6031) -> (-17.5605, -11.4252) centre (-18.8613, -9.5435) ccw projected
  line L24 (-17.5605, -11.4252) -> (-16.7665, -10.8301) projected
  arc A103 (-16.7665, -10.8301) -> (-15.3922, -12.4912) centre (1.2373, 2.6649) ccw projected
  line L25 (-15.3922, -12.4912) -> (-16.1256, -13.1597) projected
  arc A104 (-16.1256, -13.1597) -> (-16.3576, -13.4262) centre (-14.5209, -14.7901) ccw projected
  arc A105 (-16.3576, -13.4262) -> (-16.9632, -14.4022) centre (-11.3384, -17.2168) ccw projected
  arc A106 (-16.9632, -14.4022) -> (-17.7636, -16.5176) centre (-7.2503, -19.2862) ccw projected
  arc A107 (-17.7636, -16.5176) -> (-16.7142, -17.5029) centre (1.2373, 2.6649) ccw projected
  arc A108 (-16.7142, -17.5029) -> (-14.6533, -16.5713) centre (-20.1376, -7.1842) ccw projected
  arc A109 (-14.6533, -16.5713) -> (-13.7173, -15.9056) centre (-17.8156, -11.1343) ccw projected
  arc A110 (-13.7173, -15.9056) -> (-13.4658, -15.6574) centre (-15.1938, -14.1582) ccw projected
  line L26 (-13.4658, -15.6574) -> (-12.8448, -14.8835) projected
  arc A111 (-12.8448, -14.8835) -> (-11.1006, -16.1507) centre (1.2373, 2.6649) ccw projected
  line L27 (-11.1006, -16.1507) -> (-11.6447, -16.9805) projected
  arc A112 (-11.6447, -16.9805) -> (-11.8031, -17.2964) centre (-9.685, -18.1606) ccw projected
  arc A113 (-11.8031, -17.2964) -> (-12.147, -18.3923) centre (-5.9989, -19.7197) ccw projected
  arc A114 (-12.147, -18.3923) -> (-12.3961, -20.6402) centre (-1.5246, -20.7074) ccw projected
  arc A115 (-12.3961, -20.6402) -> (-11.1347, -21.3337) centre (1.2373, 2.6649) ccw projected
  arc A116 (-11.1347, -21.3337) -> (-9.3702, -19.9188) centre (-17.0167, -12.1905) ccw projected
  arc A117 (-9.3702, -19.9188) -> (-8.6292, -19.0413) centre (-13.7853, -15.4391) ccw projected
  arc A118 (-8.6292, -19.0413) -> (-8.4473, -18.7383) centre (-10.4938, -17.7159) ccw projected
  line L28 (-8.4473, -18.7383) -> (-8.0383, -17.8342) projected
  arc A119 (-8.0383, -17.8342) -> (-6.0337, -18.6279) centre (1.2373, 2.6649) ccw projected
  line L29 (-6.0337, -18.6279) -> (-6.3544, -19.5669) projected
  arc A120 (-6.3544, -19.5669) -> (-6.4292, -19.9123) centre (-4.1627, -20.2226) ccw projected
  arc A121 (-6.4292, -19.9123) -> (-6.4898, -21.0593) centre (-0.2048, -20.816) ccw projected
  arc A122 (-6.4898, -21.0593) -> (-6.1721, -23.2986) centre (4.3746, -20.6599) ccw projected
  arc A123 (-6.1721, -23.2986) -> (-4.7778, -23.6565) centre (1.2373, 2.6649) ccw projected
  arc A124 (-4.7778, -23.6565) -> (-3.4206, -21.8473) centre (-12.7488, -16.2634) ccw projected
  arc A125 (-3.4206, -21.8473) -> (-2.9211, -20.813) centre (-8.811, -18.6063) ccw projected
  arc A126 (-2.9211, -20.813) -> (-2.8203, -20.4743) centre (-5.0567, -19.9931) ccw projected
  line L30 (-2.8203, -20.4743) -> (-2.6489, -19.4969) projected
  arc A127 (-2.6489, -19.4969) -> (-0.51, -19.7671) centre (1.2373, 2.6649) ccw projected
  line L31 (-0.51, -19.7671) -> (-0.5871, -20.7565) projected
  arc A128 (-0.5871, -20.7565) -> (-0.5737, -21.1096) centre (1.6988, -20.8465) ccw projected
  arc A129 (-0.5737, -21.1096) -> (-0.3471, -22.2356) centre (5.68, -20.4369) ccw projected
  arc A130 (-0.3471, -22.2356) -> (0.5176, -24.3255) centre (10.0767, -19.1469) ccw projected
  arc A131 (0.5176, -24.3255) -> (1.957, -24.3255) centre (1.2373, 2.6649) ccw projected
  arc A132 (1.957, -24.3255) -> (2.8217, -22.2356) centre (-7.6021, -19.1469) ccw projected
  arc A133 (2.8217, -22.2356) -> (3.0483, -21.1096) centre (-3.2054, -20.4369) ccw projected
  arc A134 (3.0483, -21.1096) -> (3.0617, -20.7565) centre (0.7758, -20.8465) ccw projected
  line L32 (3.0617, -20.7565) -> (2.9846, -19.7671) projected
  arc A135 (2.9846, -19.7671) -> (5.1235, -19.4969) centre (1.2373, 2.6649) ccw projected
  line L33 (5.1235, -19.4969) -> (5.2949, -20.4743) projected
  arc A136 (5.2949, -20.4743) -> (5.3957, -20.813) centre (7.5313, -19.9931) ccw projected
  arc A137 (5.3957, -20.813) -> (5.8952, -21.8473) centre (11.2856, -18.6063) ccw projected
  arc A138 (5.8952, -21.8473) -> (7.2524, -23.6565) centre (15.2234, -16.2634) ccw projected
  arc A139 (7.2524, -23.6565) -> (8.6467, -23.2986) centre (1.2373, 2.6649) ccw projected
  arc A140 (8.6467, -23.2986) -> (8.9644, -21.0593) centre (-1.9, -20.6599) ccw projected
  arc A141 (8.9644, -21.0593) -> (8.9038, -19.9123) centre (2.6794, -20.816) ccw projected
  arc A142 (8.9038, -19.9123) -> (8.829, -19.5669) centre (6.6373, -20.2226) ccw projected
  line L34 (8.829, -19.5669) -> (8.5083, -18.6279) projected
  arc A143 (8.5083, -18.6279) -> (10.5128, -17.8342) centre (1.2373, 2.6649) ccw projected
  line L35 (10.5128, -17.8342) -> (10.9219, -18.7383) projected
  arc A144 (10.9219, -18.7383) -> (11.1038, -19.0413) centre (12.9684, -17.7159) ccw projected
  arc A145 (11.1038, -19.0413) -> (11.8448, -19.9188) centre (16.2599, -15.4391) ccw projected
  arc A146 (11.8448, -19.9188) -> (13.6093, -21.3337) centre (19.4913, -12.1905) ccw projected
  arc A147 (13.6093, -21.3337) -> (14.8707, -20.6402) centre (1.2373, 2.6649) ccw projected
  arc A148 (14.8707, -20.6402) -> (14.6216, -18.3923) centre (3.9992, -20.7074) ccw projected
  arc A149 (14.6216, -18.3923) -> (14.2777, -17.2964) centre (8.4735, -19.7197) ccw projected
  arc A150 (14.2777, -17.2964) -> (14.1193, -16.9805) centre (12.1596, -18.1606) ccw projected
  line L36 (14.1193, -16.9805) -> (13.5752, -16.1507) projected
  arc A151 (13.5752, -16.1507) -> (15.3194, -14.8835) centre (1.2373, 2.6649) ccw projected
  line L37 (15.3194, -14.8835) -> (15.9404, -15.6574) projected
  arc A152 (15.9404, -15.6574) -> (16.1919, -15.9056) centre (17.6684, -14.1582) ccw projected
  arc A153 (16.1919, -15.9056) -> (17.1279, -16.5713) centre (20.2902, -11.1343) ccw projected
  arc A154 (17.1279, -16.5713) -> (19.1888, -17.5029) centre (22.6122, -7.1842) ccw projected
  arc A155 (19.1888, -17.5029) -> (20.2382, -16.5176) centre (1.2373, 2.6649) ccw projected
  arc A156 (20.2382, -16.5176) -> (19.4378, -14.4022) centre (9.7249, -19.2862) ccw projected
  arc A157 (19.4378, -14.4022) -> (18.8322, -13.4262) centre (13.813, -17.2168) ccw projected
  arc A158 (18.8322, -13.4262) -> (18.6002, -13.1597) centre (16.9955, -14.7901) ccw projected
  line L38 (18.6002, -13.1597) -> (17.8668, -12.4912) projected
  arc A159 (17.8668, -12.4912) -> (19.2411, -10.8301) centre (1.2373, 2.6649) ccw projected
  line L39 (19.2411, -10.8301) -> (20.0351, -11.4252) projected
  arc A160 (20.0351, -11.4252) -> (20.3404, -11.6031) centre (21.3359, -9.5435) ccw projected
  arc A161 (20.3404, -11.6031) -> (21.4125, -12.0152) centre (23.1233, -5.9626) ccw projected
  arc A162 (21.4125, -12.0152) -> (23.6404, -12.405) centre (24.39, -1.5591) ccw projected
  arc A163 (23.6404, -12.405) -> (24.4117, -11.1896) centre (1.2373, 2.6649) ccw projected
  arc A164 (24.4117, -11.1896) -> (23.1104, -9.3397) centre (14.9172, -16.4858) ccw projected
  arc A165 (23.1104, -9.3397) -> (22.2811, -8.545) centre (18.3623, -13.4648) ccw projected
  arc A166 (22.2811, -8.545) -> (21.9902, -8.3445) centre (20.8413, -10.3228) ccw projected
  line L40 (21.9902, -8.3445) -> (21.1136, -7.8795) projected
  arc A167 (21.1136, -7.8795) -> (22.0315, -5.9288) centre (1.2373, 2.6649) ccw projected
  line L41 (22.0315, -5.9288) -> (22.9486, -6.3078) projected
  arc A168 (22.9486, -6.3078) -> (23.2886, -6.4041) centre (23.7406, -4.1616) ccw projected
  arc A169 (23.2886, -6.4041) -> (24.4295, -6.5366) centre (24.5813, -0.2487) ccw projected
  arc A170 (24.4295, -6.5366) -> (26.6843, -6.3601) centre (24.7131, 4.3315) ccw projected
  arc A171 (26.6843, -6.3601) -> (27.1291, -4.9911) centre (1.2373, 2.6649) ccw projected
  arc A172 (27.1291, -4.9911) -> (25.4087, -3.523) centre (19.2501, -12.4821) ccw projected
  arc A173 (25.4087, -3.523) -> (24.4078, -2.9595) centre (21.8356, -8.6992) ccw projected
  arc A174 (24.4078, -2.9595) -> (24.0761, -2.8376) centre (23.4553, -5.0394) ccw projected
  line L42 (24.0761, -2.8376) -> (23.1114, -2.6052) projected
  arc A175 (23.1114, -2.6052) -> (23.5154, -0.4875) centre (1.2373, 2.6649) ccw projected
  line L43 (23.5154, -0.4875) -> (24.4979, -0.6265) projected
  arc A176 (24.4979, -0.6265) -> (24.8511, -0.6353) centre (24.7313, 1.6492) ccw projected
  arc A177 (24.8511, -0.6353) -> (25.9892, -0.4798) centre (24.5725, 5.6483) ccw projected
  arc A178 (25.9892, -0.4798) -> (28.1293, 0.2519) centre (23.5611, 10.1173) ccw projected
  arc A179 (28.1293, 0.2519) -> (28.2196, 1.6885) centre (1.2373, 2.6649) ccw projected
  arc A180 (28.2196, 1.6885) -> (26.1881, 2.6826) centre (22.4511, -7.5266) ccw projected
  arc A181 (26.1881, 2.6826) -> (25.0786, 2.9795) centre (24.0146, -3.2196) ccw projected
  arc A182 (25.0786, 2.9795) -> (24.727, 3.015) centre (24.6733, 0.728) ccw projected
  line L44 (24.727, 3.015) -> (23.7348, 3.0002) projected
  arc A183 (23.7348, 3.0002) -> (23.5994, 5.1519) centre (1.2373, 2.6649) ccw projected
  line L45 (23.5994, 5.1519) -> (24.5857, 5.2616) projected
  arc A184 (24.5857, 5.2616) -> (24.93, 5.3409) centre (24.2458, 7.5238) ccw projected
  arc A185 (24.93, 5.3409) -> (25.9936, 5.7745) centre (23.0974, 11.3578) ccw projected
  arc A186 (25.9936, 5.7745) -> (27.8845, 7.0154) centre (21.0064, 15.4349) ccw projected
  arc A187 (27.8845, 7.0154) -> (27.6148, 8.4294) centre (1.2373, 2.6649) ccw projected
  arc A188 (27.6148, 8.4294) -> (25.3999, 8.8871) centre (24.3191, -1.9308) ccw projected
  arc A189 (25.3999, 8.8871) -> (24.2513, 8.8987) centre (24.7624, 2.6297) ccw projected
  arc A190 (24.2513, 8.8987) -> (23.902, 8.8457) centre (24.4187, 6.6172) ccw projected
  line L46 (23.902, 8.8457) -> (22.9446, 8.5846) projected
  arc A191 (22.9446, 8.5846) -> (22.2784, 10.635) centre (1.2373, 2.6649) ccw projected
  line L47 (22.2784, 10.635) -> (23.2064, 10.9865) projected
  arc A192 (23.2064, 10.9865) -> (23.5202, 11.149) centre (22.3145, 13.0932) ccw projected
  arc A193 (23.5202, 11.149) -> (24.4425, 11.8335) centre (20.2488, 16.5211) ccw projected
  arc A194 (24.4425, 11.8335) -> (25.9654, 13.5056) centre (17.2096, 19.9501) ccw projected
  arc A195 (25.9654, 13.5056) -> (25.3525, 14.8081) centre (1.2373, 2.6649) ccw projected
  arc A196 (25.3525, 14.8081) -> (23.0934, 14.7006) centre (24.7369, 3.9538) ccw projected
  arc A197 (23.0934, 14.7006) -> (21.978, 14.4262) centre (24.0321, 8.4813) ccw projected
  arc A198 (21.978, 14.4262) -> (21.6528, 14.288) centre (22.7075, 12.258) ccw projected
  line L48 (21.6528, 14.288) -> (20.7905, 13.797) projected
  arc A199 (20.7905, 13.797) -> (19.6353, 15.6173) centre (1.2373, 2.6649) ccw projected
  line L49 (19.6353, 15.6173) -> (20.4467, 16.1886) projected
  line L50 (-1.5024, 9.1136) -> (-9.0632, 16.0866) projected
  arc A200 (-8.7108, 19.4365) -> (-9.0632, 16.0866) centre (-7.6395, 17.6303) ccw projected
  arc A201 (12.2064, 18.7872) -> (-8.7108, 19.4365) centre (1.2373, 2.6649) ccw projected
  arc A202 (12.3504, 15.4219) -> (12.2064, 18.7872) centre (11.0251, 17.0509) ccw projected
  line L51 (12.3504, 15.4219) -> (4.3717, 8.9312) projected
  arc A203 (2.5774, 8.5133) -> (4.3717, 8.9312) centre (3.0465, 10.5603) ccw projected
  arc A204 (2.5774, 8.5133) -> (0.2625, 8.5852) centre (1.2373, 2.6649) ccw projected
  arc A205 (-1.5024, 9.1136) -> (0.2625, 8.5852) centre (-0.0787, 10.6573) ccw projected
  line L52 (3.333, 4.535) -> (3.9158, 3.5256) projected
  arc A206 (3.9047, 1.785) -> (3.9158, 3.5256) centre (3.4077, 2.6585) ccw projected
  line L53 (3.9047, 1.785) -> (3.322, 0.7756) projected
  arc A207 (1.8089, -0.0851) -> (3.322, 0.7756) centre (2.317, 0.782) ccw projected
  line L54 (1.8089, -0.0851) -> (0.6435, -0.0851) projected
  arc A208 (-0.8585, 0.7949) -> (0.6435, -0.0851) centre (0.1465, 0.7885) ccw projected
  line L55 (-0.8585, 0.7949) -> (-1.4412, 1.8042) projected
  arc A209 (-1.4301, 3.5449) -> (-1.4412, 1.8042) centre (-0.9331, 2.6713) ccw projected
  line L56 (-1.4301, 3.5449) -> (-0.8474, 4.5542) projected
  arc A210 (0.6657, 5.4149) -> (-0.8474, 4.5542) centre (0.1576, 4.5478) ccw projected
  line L57 (0.6657, 5.4149) -> (1.8311, 5.4149) projected
  arc A211 (3.333, 4.535) -> (1.8311, 5.4149) centre (2.3281, 4.5414) ccw projected
  arc A212 (7.0857, 1.3248) -> (7.1576, 3.6397) centre (1.2373, 2.6649) ccw projected
  arc A213 (7.686, 5.4047) -> (7.1576, 3.6397) centre (9.2297, 3.9809) ccw projected
  line L58 (7.686, 5.4047) -> (14.659, 12.9654) projected